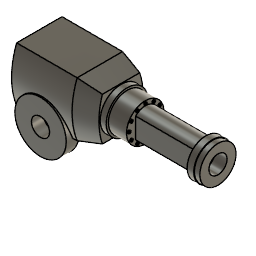
Jaw 3 (Forearm Link) (Autodesk Fusion 360 design; units mm, degrees)
part number: 2026-06-18-21-04-33-083
Autodesk Fusion 360 part; units mm, degrees
sketch "Sketch1" plane through (0, 0, 0) normal (1, 0, 0) x (0, 1, 0)
  line L0 (0, 0) -> (0, 45)
  line L1 (0, 0) -> (0, -45)
  line L2 (0, 45) -> (37.5, 45)
  line L3 (0, 45) -> (-37.5, 45)
  line L4 (0, -45) -> (37.5, -45)
  line L5 (0, -45) -> (-37.5, -45)
  arc A0 (-37.5, 45) -> (-37.5, -45) centre (79.119, 0) ccw
  arc A1 (37.5, -45) -> (37.5, 45) centre (-79.119, 0) ccw
  dimension "d1" = 37.5
  dimension "d2" = 37.5
  dimension "d3" = 37.5
  dimension "d4" = 37.5
  dimension "d5" = 125
  dimension "d6" = 125
  constraint coincident L0.start L1.start
  constraint vertical L0
  constraint parallel L0 L1
  constraint perpendicular L0 L2
  constraint perpendicular L0 L3
  constraint perpendicular L1 L4
  constraint perpendicular L1 L5
  measures "d1" distance of L0.end L2.end
  measures "d2" distance of L0.end L3.end
  measures "d3" distance of L1.end L4.end
  measures "d4" distance of L1.end L5.end
  measures "d5" radius of A0
  measures "d6" radius of A1
extrude "Extrude1" add sketch "Sketch1" along normal blind 100
extrude "Extrude2" add 1 faces at (100, -15.1807, 3.0661) along direction (1, 0, 0) blind 35 draft -15
sketch "Sketch2" plane through (135, 0, 0) normal (1, 0, 0) x (0, 1, 0)
  line L0 (-30.8786, -35.6218) -> (30.8786, -35.6218)
  arc A0 (30.8786, -35.6218) -> (30.8786, 35.6218) centre (-79.119, 0) ccw
  line L1 (30.8786, 35.6218) -> (-30.8786, 35.6218)
  arc A1 (-30.8786, 35.6218) -> (-30.8786, -35.6218) centre (79.119, 0) ccw
  circle A2 centre (0, 0) radius 34.5
  dimension "d11" = 69
  constraint coincident A2.centre origin
  measures "d11" diameter of A2
extrude "Extrude3" add sketch "Sketch2" along normal blind 10 contours A2
sketch "Sketch3" plane through (145, 0, 0) normal (1, 0, 0) x (0, 1, 0)
  circle A0 centre (0, 0) radius 34.5
  circle A1 centre (0, 0) radius 31
  dimension "d14" = 62
  constraint coincident A0.centre A1.centre
  measures "d14" diameter of A1
extrude "Extrude4" add sketch "Sketch3" along normal blind 30 contours A1
sketch "Sketch4" plane through (175, 0, 0) normal (1, 0, 0) x (0, 1, 0)
  circle A0 centre (0, 0) radius 31
  line L0 (0, 0) -> (27, 0)
  circle A1 centre (27, 0) radius 2.5
  circle A2 centre (27, 0) radius 1.5
  dimension "d17" = 27
  dimension "d18" = 5
  dimension "d19" = -1
  constraint coincident A0.centre L0.start
  constraint horizontal L0
  constraint coincident L0.end A1.centre
  measures "d17" distance of A0.centre L0.end
  measures "d18" diameter of A1
extrude "Extrude5" add sketch "Sketch4" along normal blind 1 contours A1
pattern_circular "C-Pattern1" count 12 over 360 about axis through (175, 0, 0) along (1, 0, 0) of "Extrude5"
sketch "Sketch5" plane through (175, 0, 0) normal (1, 0, 0) x (0, 1, 0)
  circle A0 centre (13.5, -23.3827) radius 2.5
  circle A1 centre (-13.5, -23.3827) radius 2.5
  circle A2 centre (-27, 0) radius 2.5
  circle A3 centre (-13.5, 23.3827) radius 2.5
  circle A4 centre (13.5, 23.3827) radius 2.5
  circle A5 centre (27, 0) radius 2.5
  circle A6 centre (0, 0) radius 31
  circle A7 centre (23.3827, 13.5) radius 2.5
  circle A8 centre (0, 27) radius 2.5
  circle A9 centre (-23.3827, 13.5) radius 2.5
  circle A10 centre (-23.3827, -13.5) radius 2.5
  circle A11 centre (0, -27) radius 2.5
  circle A12 centre (23.3827, -13.5) radius 2.5
  line L0 (16, 0) -> (16, 17)
  line L1 (16, 0) -> (16, -17)
  line L2 (-16, 0) -> (-16, 17)
  line L3 (-16, 0) -> (-16, -17)
  arc A13 (-16, -17) -> (16, -17) centre (0, -1.9003) ccw
  arc A14 (16, 17) -> (-16, 17) centre (0, 1.9003) ccw
  dimension "d32" = 22
  dimension "d33" = 17
  dimension "d34" = 17
  measures "d32" radius of A13
  measures "d33" distance of L0.start L1.end
  measures "d34" distance of L0.start L0.end
extrude "Extrude6" add sketch "Sketch5" along normal blind 100 contours L0 L1 L2 L3 A13 A14
sketch "Sketch6" plane through (275, 0, 0) normal (1, 0, 0) x (0, 1, 0)
  line L0 (16, -17) -> (16, 17)
  arc A0 (16, 17) -> (-16, 17) centre (0, 1.9003) ccw
  line L1 (-16, 17) -> (-16, -17)
  arc A1 (-16, -17) -> (16, -17) centre (0, -1.9003) ccw
  circle A2 centre (0, 0) radius 31
  dimension "d37" = 62
  constraint coincident A2.centre origin
  measures "d37" diameter of A2
extrude "Extrude7" add sketch "Sketch6" along normal blind 10 contours L0 A0 L1 A1 | A2
sketch "Sketch7" plane through (285, 0, 0) normal (1, 0, 0) x (0, 1, 0)
  circle A0 centre (0, 0) radius 31
  circle A1 centre (0, 0) radius 30
  dimension "d40" = -1
extrude "Extrude8" add sketch "Sketch7" along normal blind 1
sketch "Sketch8" plane through (285, 0, 0) normal (1, 0, 0) x (0, 1, 0)
  circle A0 centre (0, 0) radius 30
  circle A1 centre (0, 0) radius 31
  dimension "d43" = 62
  constraint coincident A0.centre A1.centre
  measures "d43" diameter of A1
extrude "Extrude9" add sketch "Sketch8" along normal blind 10 contours A0
ref_plane "WorkPlane1" through (0, -37.5, 45) normal (0, -1, 0) x (1, 0, 0)
sketch "Sketch9" plane through (0, -37.5, 0) normal (0, -1, 0) x (-1, 0, 0)
  circle A0 centre (-50, 45) radius 42.5
  dimension "d46" = 85
  measures "d46" diameter of A0
extrude "Extrude10" add sketch "Sketch9" along normal mid plane 21
sketch "Sketch10" plane through (0, -27, 0) normal (0, 1, 0) x (-1, 0, 0)
  line L0 (-7.5, -45) -> (-92.5, -45)
  arc A0 (-92.5, -45) -> (-7.5, -45) centre (-50, -45) ccw
  line L1 (-50, -45) -> (-50, -75)
  line L2 (-70, -45) -> (-70, -77.2846)
  line L3 (-30, -45) -> (-30, -77.2846)
  arc A1 (-70, -77.2846) -> (-30, -77.2846) centre (-50, -54.924) ccw
  dimension "d49" = 30
  dimension "d50" = 20
  dimension "d51" = -20
  dimension "d52" = 30
  constraint coincident A0.centre L1.start
  constraint perpendicular L0 L1
  measures "d49" distance of A0.centre L1.end
  measures "d52" radius of A1
extrude "Extrude11" add sketch "Sketch10" along normal blind 35 contours L0 L2 L3 A1
sketch "Sketch11" plane through (70, 0, 0) normal (1, 0, 0) x (0, 1, 0)
  line L0 (-27, -45) -> (-27, -77.2846)
  line L1 (-27, -77.2846) -> (8, -77.2846)
  line L2 (8, -77.2846) -> (8, -45)
  line L3 (8, -45) -> (-27, -45)
  line L4 (8, -45) -> (33, -45)
  line L5 (8, -45) -> (8, -87)
  arc A0 (8, -87) -> (33, -45) centre (-21.8393, -40.7981) ccw
  dimension "d55" = 25
  dimension "d56" = 42
  dimension "d57" = 55
  constraint coincident L2.end L3.start
  constraint perpendicular L2 L4
  constraint perpendicular L1 L5
  measures "d55" distance of L2.end L4.end
  measures "d56" distance of L2.end L5.end
  measures "d57" radius of A0
extrude "Extrude12" add sketch "Sketch11" against normal blind 40 contours L2 L4 L5 A0
extrude "Extrude13" cut 1 faces at (33.5817, 8, -83.0165) along direction (0, 1, 0) blind 25
sketch "Sketch12" plane through (295, 0, 0) normal (1, 0, 0) x (0, 1, 0)
  circle A0 centre (0, 0) radius 30
  circle A1 centre (0, 0) radius 15
  dimension "d62" = 30
  constraint coincident A0.centre A1.centre
  measures "d62" diameter of A1
extrude "Extrude14" cut sketch "Sketch12" against normal blind 20 contours A1
sketch "Sketch13" plane through (0, -48, 0) normal (0, -1, 0) x (1, 0, 0)
  circle A0 centre (50, -45) radius 42.5
  circle A1 centre (50, -45) radius 15
  dimension "d65" = 30
  constraint concentric A0 A1
  measures "d65" diameter of A1
extrude "Extrude15" cut sketch "Sketch13" against normal blind 20 contours A1
equation "d47 = ( 21 / 2 ) * 1 mm"
